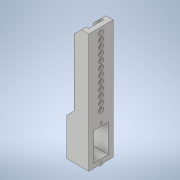
# Autodesk Inventor part: TopRearLeg4
Saved by Autodesk Inventor 2020 (Build 240168000, 168)
## iProperties
Created: 2019-03-31
Part Number: TopRearLeg4
Material: Generic
Document SubType Name: Modeling
Designer: cnam
Density: 1 g/cm^3
Appearance: Default
Author: cnam
Autodesk Inventor part; units mm, degrees
ref_plane "YZ Plane" through (0, 0, 0) normal (1, 0, 0) x (0, 1, 0)
ref_plane "XZ Plane" through (0, 0, 0) normal (0, 1, 0) x (-1, 0, 0)
ref_plane "XY Plane" through (0, 0, 0) normal (0, 0, 1) x (1, 0, 0)
sketch "Sketch1" plane through (0, 0, 0) normal (1, 0, 0) x (0, 1, 0)
  line L0 (47.75, -10) -> (-47.75, -10)
  line L1 (-47.75, -10) -> (-47.75, 10)
  line L2 (-47.75, 10) -> (47.75, 10)
  line L3 (47.75, 10) -> (47.75, -10)
  line L4 (47.75, -10) -> (-47.75, 10) construction
  line L5 (-47.75, -10) -> (47.75, 10) construction
  circle A0 centre (40.75, 0) radius 2
  circle A1 centre (-4.25, 0) radius 2
  line L6 (18.25, 25.1028) -> (18.25, -34.7635) construction
  line L7 (-1.75, 23.8417) -> (-1.75, -36.7999) construction
  circle A2 centre (20.75, 0) radius 2
  circle A3 centre (-24.25, 0) radius 2
  line L8 (-41.75, 23.8417) -> (-41.75, -30.9921) construction
  circle A4 centre (34.0833, 0) radius 2
  circle A5 centre (27.4167, 0) radius 2
  circle A6 centre (-10.9167, 0) radius 2
  circle A7 centre (-17.5833, 0) radius 2
  point P0 (0, 0)
  dimension "d1" = 20
  dimension "d4" = 4
  dimension "d5" = 7
  dimension "d6" = 45
  dimension "d7" = 22.5
  dimension "d8" = 20
  dimension "d9" = 22.5
  dimension "d10" = 22.5
  dimension "d11" = 60
  dimension "d18" = 6.6667
  dimension "d25" = 6.6667
  dimension "d30" = 6
  constraints: 18 end point, 8 centre point, 3 equal radius, 3 horizontal, 3 vertical, 2 midpoint, 2 parallel, 1 perpendicular, 8 other
  measures "d1" distance of L2.end L0.start
  measures "d4" diameter of A0
  measures "d5" distance from line of L3 A0.centre
  measures "d6" distance of A1.centre A0.centre
  measures "d7" distance from line of L6 A0.centre
  measures "d8" distance between parallel lines of L6 L7
  measures "d9" distance from line of L7 A2.centre
  measures "d10" distance from line of L7 A3.centre
  measures "d11" distance between parallel lines of L8 L6
  measures "d18" distance of A0.centre A4.centre
  measures "d25" distance of A1.centre A6.centre
  measures "d30" distance between parallel lines of L8 L1
extrude "Extrusion1" add sketch "Sketch1" along normal blind 4
sketch "Sketch2" plane through (0, 0, 0) normal (1, 0, 0) x (0, 1, 0)
  line L0 (-41.75, 22.3574) -> (-41.75, -36.9148) construction
  circle A0 centre (-17.5833, 0) radius 2 projected
  circle A1 centre (-10.9167, 0) radius 2 projected
  circle A2 centre (27.4167, 0) radius 2 projected
  circle A3 centre (34.0833, 0) radius 2 projected
  circle A4 centre (-24.25, 0) radius 2 projected
  circle A5 centre (20.75, 0) radius 2 projected
  circle A6 centre (-4.25, 0) radius 2 projected
  circle A7 centre (40.75, 0) radius 2 projected
  line L1 (-47.75, -10) -> (47.75, -10) projected
  line L2 (47.75, -10) -> (47.75, 10) projected
  line L3 (47.75, 10) -> (-47.75, 10) projected
  line L4 (-47.75, 10) -> (-47.75, -10) projected
  line L5 (47.75, 0) -> (-47.75, 0) construction
  line L6 (-47.75, -10) -> (-47.75, 10) projected
  line L7 (-59.75, -6.125) -> (-36.75, -6.125)
  line L8 (-36.75, -6.125) -> (-36.75, 6.125)
  line L9 (-36.75, 6.125) -> (-59.75, 6.125)
  line L10 (-59.75, 6.125) -> (-59.75, -6.125)
  line L11 (-59.75, -6.125) -> (-36.75, 6.125) construction
  line L12 (-36.75, -6.125) -> (-59.75, 6.125) construction
  line L13 (-47.75, -10) -> (-63.625, -10)
  line L14 (-63.625, -10) -> (-63.625, 10)
  line L15 (-63.625, 10) -> (-47.75, 10)
  line L16 (-47.75, 10) -> (-47.75, -10)
  line L17 (-32.875, -10) -> (-32.875, 10)
  point P0 (0, 0)
  point P1 (-48.25, 0)
  dimension "d33" = 6
  dimension "d34" = 12.25
  dimension "d35" = 23
  dimension "d36" = 5
  dimension "d37" = 3.875
  dimension "d38" = 3.875
  dimension "d39" = 3.875
  constraints: 26 end point, 4 midpoint, 4 parallel, 3 perpendicular, 3 point on line, 2 horizontal, 1 vertical
  measures "d33" distance between parallel lines of L4 L0
  measures "d34" distance of L7.end L8.end
  measures "d35" distance of L7.start L7.end
  measures "d36" distance between parallel lines of L0 L8
  measures "d37" distance between parallel lines of L15 L9
  measures "d38" distance between parallel lines of L14 L10
  measures "d39" distance between parallel lines of L8 L17
extrude "Extrusion2" cut sketch "Sketch2" along normal blind 20 contours L7 L10 L9 L4 | L4 L9 L8 L7
sketch "Sketch3" plane through (0, 0, 0) normal (-1, 0, 0) x (0, 0, 1)
  line L0 (-10, -47.75) -> (-6.125, -47.75) projected
  line L1 (-10, -47.75) -> (-6.125, -47.75)
  line L2 (6.125, -47.75) -> (10, -47.75) projected
  line L3 (10, -47.75) -> (6.125, -47.75)
  line L4 (6.125, -36.75) -> (6.125, -47.75) projected
  line L5 (6.125, -47.75) -> (10, -47.75) projected
  line L6 (10, -47.75) -> (10, 47.75) projected
  line L7 (10, 47.75) -> (-10, 47.75) projected
  line L8 (-10, 47.75) -> (-10, -47.75) projected
  line L9 (-10, -47.75) -> (-6.125, -47.75) projected
  line L10 (-6.125, -47.75) -> (-6.125, -36.75) projected
  line L11 (-6.125, -36.75) -> (6.125, -36.75) projected
  circle A0 centre (0, -17.5833) radius 2 projected
  circle A1 centre (0, -10.9167) radius 2 projected
  circle A2 centre (0, 27.4167) radius 2 projected
  circle A3 centre (0, 34.0833) radius 2 projected
  circle A4 centre (0, -24.25) radius 2 projected
  circle A5 centre (0, 20.75) radius 2 projected
  circle A6 centre (0, -4.25) radius 2 projected
  circle A7 centre (0, 40.75) radius 2 projected
  line L12 (-6.125, -36.75) -> (6.125, -36.75)
  line L13 (6.125, -36.75) -> (6.125, -59.75)
  line L14 (6.125, -59.75) -> (-6.125, -59.75)
  line L15 (-6.125, -59.75) -> (-6.125, -36.75)
  line L16 (-10, 47.75) -> (-10, -47.75) projected
  line L17 (-10, -32.875) -> (10, -32.875)
  line L18 (10, -32.875) -> (10, -63.625)
  line L19 (10, -63.625) -> (-10, -63.625)
  line L20 (-10, -63.625) -> (-10, -32.875)
  point P0 (0, 0)
  dimension "d44" = 23
  dimension "d45" = 3.875
  dimension "d46" = 3.875
  dimension "d47" = 3.875
  constraints: 20 end point, 5 equal length, 3 horizontal, 2 perpendicular, 1 point on line
  measures "d44" distance of L12.end L13.end
  measures "d45" distance between parallel lines of L12 L17
  measures "d46" distance between parallel lines of L19 L14
  measures "d47" distance between parallel lines of L18 L13
extrude "Extrusion4" add sketch "Sketch3" along normal blind 20 contours L8 L17 L6 L2 L4 L11 L10 L0 | L0 L15 L14 L13 L2 L18 L19 L20
sketch "Sketch5" plane through (0, 0, 0) normal (1, 0, 0) x (0, 0, -1)
  line L0 (-6.125, -47.75) -> (-10, -47.75) projected
  line L1 (-10, -63.625) -> (-10, -47.75) projected
  line L2 (10, -63.625) -> (-10, -63.625) projected
  line L3 (10, -47.75) -> (10, -63.625) projected
  line L4 (10, -47.75) -> (6.125, -47.75) projected
  line L5 (6.125, -47.75) -> (6.125, -59.75) projected
  line L6 (6.125, -59.75) -> (-6.125, -59.75) projected
  line L7 (-6.125, -59.75) -> (-6.125, -47.75) projected
  point P0 (0, 0)
extrude "Extrusion5" add sketch "Sketch5" along normal blind 4
sketch "Sketch6" plane through (0, 0, 0) normal (-1, 0, 0) x (0, 0, 1)
  line L0 (-10, -32.875) -> (10, -32.875) projected
  line L1 (10, -32.875) -> (10, 47.75) projected
  line L2 (10, 47.75) -> (-10, 47.75) projected
  line L3 (-10, 47.75) -> (-10, -32.875) projected
  circle A0 centre (0, -17.5833) radius 2 projected
  circle A1 centre (0, -10.9167) radius 2 projected
  circle A2 centre (0, 27.4167) radius 2 projected
  circle A3 centre (0, 34.0833) radius 2 projected
  circle A4 centre (0, -24.25) radius 2 projected
  circle A5 centre (0, 20.75) radius 2 projected
  circle A6 centre (0, -4.25) radius 2 projected
  circle A7 centre (0, 40.75) radius 2 projected
  circle A8 centre (0, -30.375) radius 0.875
  point P0 (0, 0)
  dimension "d52" = 2.5
  dimension "d53" = 1.75
  constraints: 1 centre point
  measures "d52" distance from line of L0 A8.centre
  measures "d53" diameter of A8
extrude "Extrusion6" cut sketch "Sketch6" against normal blind 4 contours A8
sketch "Sketch8" plane through (4, 47.75, -10) normal (0, 0, -1) x (-1, 0, 0)
  line L0 (24, -84.5) -> (0, -84.5) projected
  line L1 (4, 0) -> (4, -80.625) projected
  line L2 (4, 0) -> (0, 0) projected
  line L3 (0, -111.375) -> (0, 0) projected
  line L4 (0, -111.375) -> (24, -111.375) projected
  line L5 (24, -80.625) -> (24, -111.375) projected
  line L6 (4, -80.625) -> (24, -80.625) projected
  line L7 (4, -80.625) -> (4, 0) projected
  line L8 (4, 0) -> (4, -80.625) projected
  line L9 (24, -80.625) -> (4, 0)
  point P0 (4, -47.75)
  constraints: 2 end point
extrude "Extrusion8" add sketch "Sketch8" against normal blind 3 contours L6 L1 L9
mirror "Mirror2" about plane through (0, 0, 0) normal (0, 0, 1) of "Extrusion8"
sketch "Sketch9" plane through (4, 0, 0) normal (1, 0, 0) x (0, 0, -1)
  circle A0 centre (0, -30.375) radius 0.875 projected
  line L0 (10, -63.625) -> (10, 47.75) projected
  line L1 (10, 47.75) -> (-10, 47.75) projected
  line L2 (-10, 47.75) -> (-10, -63.625) projected
  line L3 (-10, -63.625) -> (10, -63.625) projected
  line L4 (6.125, -36.75) -> (6.125, -59.75) projected
  line L5 (6.125, -59.75) -> (-6.125, -59.75) projected
  line L6 (-6.125, -59.75) -> (-6.125, -36.75) projected
  line L7 (-6.125, -36.75) -> (6.125, -36.75) projected
  circle A1 centre (0, 40.75) radius 2 projected
  circle A2 centre (0, -4.25) radius 2 projected
  circle A3 centre (0, 20.75) radius 2 projected
  circle A4 centre (0, -24.25) radius 2 projected
  circle A5 centre (0, 34.0833) radius 2 projected
  circle A6 centre (0, 27.4167) radius 2 projected
  circle A7 centre (0, -10.9167) radius 2 projected
  circle A8 centre (0, -17.5833) radius 2 projected
  point P0 (0, 0)
sketch "Sketch10" plane through (0, 0, 0) normal (-1, 0, 0) x (0, 0, 1)
  line L0 (-3.7215, 44.8818) -> (4.317, 44.8818)
  line L1 (4.317, 44.8818) -> (4.317, -27.7627)
  line L2 (4.317, -27.7627) -> (-3.7215, -27.7627)
  line L3 (-3.7215, -27.7627) -> (-3.7215, 44.8818)
  point P0 (0, 0)
  constraints: 8 end point, 2 parallel, 1 horizontal, 1 perpendicular
extrude "Extrusion9" add sketch "Sketch10" against normal blind 4
sketch "Sketch11" plane through (0, 0, 0) normal (-1, 0, 0) x (0, 0, 1)
  circle A0 centre (0, -30.375) radius 0.875 projected
  line L0 (7, -32.875) -> (7, 47.75) projected
  line L1 (7, 47.75) -> (-7, 47.75) projected
  line L2 (-7, 47.75) -> (-7, -32.875) projected
  line L3 (-7, -32.875) -> (7, -32.875) projected
  arc A1 (2, -30.375) -> (-2, -30.375) centre (0, -30.375) ccw
  line L4 (-7, -32.875) -> (7, -32.875) projected
  line L5 (-0.875, -30.375) -> (0.875, -30.375)
  line L6 (2, -30.375) -> (2, -32.875)
  line L7 (2, -32.875) -> (-2, -32.875)
  line L8 (-2, -32.875) -> (-2, -30.375)
  point P0 (0, 0)
  point P1 (-2, -32.875)
  dimension "d68" = 4
  constraints: 8 end point, 4 point on circle, 2 parallel, 1 centre point, 1 coincident, 1 horizontal, 1 perpendicular, 1 point on line
  measures "d68" diameter of A1
extrude "Extrusion10" add sketch "Sketch11" along normal blind 20 contours L3 L8 A1 L6
sketch "Sketch12" plane through (0, 0, 0) normal (-1, 0, 0) x (0, 0, 1)
  line L0 (2, -30.375) -> (2, -32.875) projected
  line L1 (2, -32.875) -> (7, -32.875) projected
  line L2 (7, -32.875) -> (7, 47.75) projected
  line L3 (7, 47.75) -> (-7, 47.75) projected
  line L4 (-7, 47.75) -> (-7, -32.875) projected
  line L5 (-7, -32.875) -> (-2, -32.875) projected
  line L6 (-2, -32.875) -> (-2, -30.375) projected
  arc A0 (2, -30.375) -> (-2, -30.375) centre (0, -30.375) ccw projected
  point P0 (0, 0)
  point P1 (0, 44.75)
  point P2 (0, 39.75)
  point P3 (0, 34.75)
  point P4 (0, 29.75)
  point P5 (0, 24.75)
  point P6 (0, 19.75)
  point P7 (0, 14.75)
  point P8 (0, 9.75)
  point P9 (0, 4.75)
  point P10 (0, -0.25)
  point P11 (0, -5.25)
  point P12 (0, -10.25)
  point P13 (0, -15.25)
  point P14 (0, -20.25)
  point P15 (0, -25.25)
  dimension "d74" = 5
  constraints: 1 vertical, 14 other
  measures "d74" distance of point (0, 44.75) point (0, 39.75)
hole "Hole1" at (0, 44.75, 0) at (0, 39.75, 0) at (0, 34.75, 0) at (0, 29.75, 0) at (0, 24.75, 0) at (0, 19.75, 0) at (0, 14.75, 0) at (0, 9.75, 0) at (0, 4.75, 0) at (0, -0.25, 0) at (0, -5.25, 0) at (0, -10.25, 0) at (0, -15.25, 0) at (0, -20.25, 0) at (0, -25.25, 0) direction (1, 0, 0) diameter 4 end through all
sketch "Sketch13" plane through (-20, 0, 0) normal (-1, 0, 0) x (0, 0, 1)
  line L0 (-19.5017, -86.8207) -> (19.9399, -86.8207)
  line L1 (19.9399, -86.8207) -> (19.9399, 61.3045)
  line L2 (19.9399, 61.3045) -> (-19.5017, 61.3045)
  line L3 (-19.5017, 61.3045) -> (-19.5017, -86.8207)
  point P0 (0, 0)
  constraints: 8 end point, 2 parallel, 1 horizontal, 1 perpendicular
extrude "Extrusion11" cut sketch "Sketch13" against normal blind 6
sketch "Sketch14" plane through (-14, 0, 0) normal (-1, 0, 0) x (0, 0, 1)
  line L0 (6.125, -59.75) -> (6.125, -36.75) projected
  line L1 (6.125, -59.75) -> (6.125, -36.75) projected
  line L2 (6.125, -48.25) -> (-6.125, -48.25)
  line L3 (-6.125, -36.75) -> (-6.125, -59.75) projected
  point P0 (0, 0)
  constraints: 2 end point, 2 midpoint
surface extrude "ExtrusionSrf1" sketch "Sketch14" against normal mid plane 50 shown no curves L2
mirror "Mirror3" about plane through (-14, -48.25, 6.125) normal (0, -1, 0) of "Extrusion10"
sketch "Sketch15" plane through (-20, -66.125, -2) normal (-1, 0, 0) x (0, 0, 1)
  circle A0 centre (2, 0) radius 0.875 projected
  line L0 (0, 0) -> (0, 2.5) projected
  arc A1 (0, 0) -> (4, 0) centre (2, 0) ccw projected
  line L1 (4, 2.5) -> (4, 0) projected
  line L2 (0, 2.5) -> (4, 2.5) projected
  circle A2 centre (2, 0) radius 0.875 projected
  point P0 (2, 66.125)
extrude "Extrusion12" cut sketch "Sketch15" against normal up to surface (6 mm away) contours A0 | L0 L2 L1 A1
sketch "Sketch16" plane through (0, -66.125, -2) normal (1, 0, 0) x (0, 0, -1)
  line L0 (0, 0) -> (0, 2.5) projected
  line L1 (-4, 2.5) -> (0, 2.5) projected
  line L2 (-4, 2.5) -> (-4, 0) projected
  arc A0 (-4, 0) -> (0, 0) centre (-2, 0) ccw projected
  circle A1 centre (-2, 0) radius 0.875 projected
  point P0 (-2, 66.125)
extrude "Extrusion13" add sketch "Sketch16" along normal up to surface (4 mm away)
chamfer "Chamfer1" distance 16 angle 45 2 edges at (-14, -8.6875, -8.5) (-14, -8.6875, 8.5)
sketch "Sketch17" plane through (-14, 0, 0) normal (-1, 0, 0) x (0, 0, 1)
  circle A0 centre (0, -66.125) radius 0.875 projected
  circle A1 centre (0, -30.375) radius 0.875 projected
  line L0 (7, -24.6875) -> (10, -24.6875) projected
  line L1 (7, -32.875) -> (7, -24.6875) projected
  line L2 (2, -32.875) -> (7, -32.875) projected
  line L3 (2, -30.375) -> (2, -32.875) projected
  arc A2 (2, -30.375) -> (-2, -30.375) centre (0, -30.375) ccw projected
  line L4 (-2, -32.875) -> (-2, -30.375) projected
  line L5 (-7, -32.875) -> (-2, -32.875) projected
  line L6 (-7, -24.6875) -> (-7, -32.875) projected
  line L7 (-10, -24.6875) -> (-7, -24.6875) projected
  line L8 (-10, -63.625) -> (-10, -24.6875) projected
  line L9 (-2, -63.625) -> (-10, -63.625) projected
  line L10 (-2, -66.125) -> (-2, -63.625) projected
  arc A3 (-2, -66.125) -> (2, -66.125) centre (0, -66.125) ccw projected
  line L11 (2, -63.625) -> (2, -66.125) projected
  line L12 (10, -63.625) -> (2, -63.625) projected
  line L13 (10, -24.6875) -> (10, -63.625) projected
  line L14 (6.125, -36.75) -> (-6.125, -36.75) projected
  line L15 (6.125, -59.75) -> (6.125, -36.75) projected
  line L16 (-6.125, -59.75) -> (6.125, -59.75) projected
  line L17 (-6.125, -36.75) -> (-6.125, -59.75) projected
  line L18 (-7, -24.6875) -> (-7, -32.875) projected
  line L19 (-7, -32.875) -> (-26.1953, -32.875)
  line L20 (-26.1953, -32.875) -> (-26.1953, 59.8507)
  line L21 (-26.1953, 59.8507) -> (-7, 59.8507)
  line L22 (-7, 59.8507) -> (-7, -32.875)
  line L23 (2, -32.875) -> (7, -32.875) projected
  line L24 (7, -32.875) -> (27.7212, -32.875)
  line L25 (27.7212, -32.875) -> (27.7212, 59.8507)
  line L26 (27.7212, 59.8507) -> (7, 59.8507)
  line L27 (7, 59.8507) -> (7, -32.875)
  point P0 (0, 0)
  constraints: 16 end point, 4 parallel, 2 horizontal, 2 perpendicular, 1 point on line
extrude "Extrusion14" cut sketch "Sketch17" against normal up to surface (14 mm away) contours L27 L26 L25 L24 L13 L0 | L0 L13 L24 L1 | L19 L8 L7 L6 | L7 L8 L19 L20 L21 L22
sketch "Sketch18" plane through (0, 47.75, 10) normal (0, 0, 1) x (1, 0, 0)
  line L0 (0, 0) -> (0, -80.625) projected
  line L1 (0, -80.625) -> (-14, -80.625) projected
  line L2 (-14, -80.625) -> (-14, -111.375) projected
  line L3 (4, -111.375) -> (-14, -111.375) projected
  line L4 (4, 0) -> (4, -111.375) projected
  line L5 (0, 0) -> (4, 0) projected
  line L6 (-14, -80.625) -> (0, -80.625) projected
  line L7 (-14, -80.625) -> (0, -66.625)
  point P0 (0, -47.75)
  dimension "d101" = 45
  constraints: 2 end point, 1 point on line
  measures "d101" angle of L1 L7
extrude "Extrusion15" add sketch "Sketch18" against normal blind 4 contours L0 L1 L7
sketch "Sketch19" plane through (0, 0, 0) normal (-1, 0, 0) x (0, 0, 1)
  line L0 (10, 47.75) -> (10, -63.625) projected
  line L1 (6, -32.875) -> (2, -32.875) projected
  line L2 (10, 47.75) -> (6, 47.75)
  line L3 (6, 47.75) -> (6, -32.875)
  line L4 (6, -32.875) -> (10, -32.875)
  line L5 (10, -32.875) -> (10, 47.75)
  point P0 (0, 0)
  constraints: 8 end point, 2 parallel, 1 horizontal, 1 perpendicular
extrude "Extrusion16" add sketch "Sketch19" along normal blind 8
chamfer "Chamfer2" distance 8 angle 45 1 edges at (-8, 47.75, 8)
mirror "Mirror4" about plane through (0, 0, 0) normal (0, 0, 1) of "Extrusion15", "Extrusion16", "Chamfer2"
fillet "Fillet4" radius 4 2 edges at (2, 47.75, 10) (2, 47.75, -10)
fillet "Fillet5" radius 4 2 edges at (-8, 39.75, -8) (-8, 39.75, 8)
sketch "Sketch20" plane through (-14, 0, 0) normal (-1, 0, 0) x (0, 0, 1)
  line L0 (6.125, -36.75) -> (-6.125, -36.75) projected
  line L1 (-6.125, -59.75) -> (6.125, -59.75) projected
  point P0 (0, 0)
  point P1 (0, -34.25)
  point P2 (0, -62.25)
  dimension "d111" = 2.5
  dimension "d112" = 2.5
  measures "d111" distance from line of L0 point (0, -34.25)
  measures "d112" distance from line of point (0, -62.25) L1
hole "Hole2" at (-14, -34.25, 0) at (-14, -62.25, 0) direction (1, 0, 0) diameter 1.75 end through all
sketch "Sketch21" plane through (-14, 0, 0) normal (-1, 0, 0) x (0, 0, 1)
  circle A0 centre (0, -34.25) radius 0.875 projected
  circle A1 centre (0, -62.25) radius 0.875 projected
  line L0 (10, -32.875) -> (6, -32.875) projected
  line L1 (6, -32.875) -> (2, -32.875) projected
  line L2 (2, -30.375) -> (2, -32.875) projected
  arc A2 (2, -30.375) -> (-2, -30.375) centre (0, -30.375) ccw projected
  line L3 (-2, -32.875) -> (-2, -30.375) projected
  line L4 (-2, -32.875) -> (-6, -32.875) projected
  line L5 (-6, -32.875) -> (-10, -32.875) projected
  line L6 (-10, -63.625) -> (-10, -32.875) projected
  line L7 (-2, -63.625) -> (-10, -63.625) projected
  line L8 (-2, -66.125) -> (-2, -63.625) projected
  arc A3 (-2, -66.125) -> (2, -66.125) centre (0, -66.125) ccw projected
  line L9 (2, -63.625) -> (2, -66.125) projected
  line L10 (10, -63.625) -> (2, -63.625) projected
  line L11 (10, -32.875) -> (10, -63.625) projected
  line L12 (6.125, -36.75) -> (-6.125, -36.75) projected
  line L13 (6.125, -59.75) -> (6.125, -36.75) projected
  line L14 (-6.125, -59.75) -> (6.125, -59.75) projected
  line L15 (-6.125, -36.75) -> (-6.125, -59.75) projected
  circle A4 centre (0, -30.375) radius 0.875 projected
  circle A5 centre (0, -66.125) radius 0.875 projected
  line L16 (-2, -63.625) -> (2, -63.625)
  line L17 (6, -32.875) -> (2, -32.875) projected
  line L18 (2, -32.875) -> (-2, -32.875)
  point P0 (0, 0)
  constraints: 4 end point, 1 collinear, 1 horizontal
extrude "Extrusion17" cut sketch "Sketch21" against normal up to surface (14 mm away) contours L18 L3 A2 L2 | L9 A3 L8 L16
sketch "Sketch22" plane through (0, -66.125, -2) normal (-1, 0, 0) x (0, 0, 1)
  circle A0 centre (2, 0) radius 0.875 projected
  line L0 (4, 2.5) -> (0, 2.5) projected
  line L1 (0, 0) -> (0, 2.5) projected
  arc A1 (0, 0) -> (4, 0) centre (2, 0) ccw projected
  line L2 (4, 2.5) -> (4, 0) projected
  point P0 (2, 66.125)
extrude "Extrusion18" cut sketch "Sketch22" against normal blind 10 contours A0 | L2 A1 L1 L0
sketch "Sketch23" plane through (0, 0, 0) normal (-1, 0, 0) x (0, 0, 1)
  circle A0 centre (0, -30.375) radius 0.875 projected
  point P0 (0, 0)
extrude "Extrusion19" add sketch "Sketch23" against normal blind 4
sketch "Sketch24" plane through (-14, 0, 0) normal (-1, 0, 0) x (0, 0, 1)
  line L0 (10, -63.625) -> (-10, -63.625) projected
  line L1 (10, -32.875) -> (10, -63.625) projected
  line L2 (10, -32.875) -> (6, -32.875) projected
  line L3 (6, -32.875) -> (-6, -32.875) projected
  line L4 (-6, -32.875) -> (-10, -32.875) projected
  line L5 (-10, -63.625) -> (-10, -32.875) projected
  circle A0 centre (0, -34.25) radius 0.875 projected
  circle A1 centre (0, -62.25) radius 0.875 projected
  line L6 (6.125, -36.75) -> (-6.125, -36.75) projected
  line L7 (6.125, -59.75) -> (6.125, -36.75) projected
  line L8 (-6.125, -59.75) -> (6.125, -59.75) projected
  line L9 (-6.125, -36.75) -> (-6.125, -59.75) projected
  circle A2 centre (0, -34.25) radius 0.875 projected
  circle A3 centre (0, -34.25) radius 2.5
  circle A4 centre (0, -62.25) radius 2.5
  point P0 (0, 0)
  point P1 (-2.0879, -32.875)
  point P2 (2.0879, -32.875)
  point P3 (-2.0879, -63.625)
  point P4 (2.0879, -63.625)
  constraints: 2 centre point, 2 coincident
extrude "Extrusion20" add sketch "Sketch24" against normal up to surface (18 mm away) contours A4 L0 | L3 A3 picked at (-0.2038, -63.9747) picked at (-0.2038, -32.2127)
sketch "Sketch25" plane through (0, 0, 0) normal (-1, 0, 0) x (0, 0, 1)
  circle A0 centre (0, 34.75) radius 2 projected
  circle A1 centre (0, 39.75) radius 2 projected
  circle A2 centre (0, 44.75) radius 2 projected
  point P0 (0, 0)
extrude "Extrusion21" add sketch "Sketch25" against normal up to surface (4 mm away)
sketch "Sketch26" plane through (0, 0, 0) normal (-1, 0, 0) x (0, 0, 1)
  line L0 (-17.4187, 33.75) -> (21.8321, 33.75)
  line L1 (21.8321, 33.75) -> (21.8321, 58.5819)
  line L2 (21.8321, 58.5819) -> (-17.4187, 58.5819)
  line L3 (-17.4187, 58.5819) -> (-17.4187, 33.75)
  circle A0 centre (0, 29.75) radius 2 projected
  point P0 (0, 0)
  dimension "d130" = 4
  constraints: 8 end point, 2 parallel, 1 horizontal, 1 perpendicular
  measures "d130" distance from line of L0 A0.centre
extrude "Extrusion22" cut sketch "Sketch26" along normal blind 10 and the other way blind 5 contours L3 L2 L1 L0
chamfer "Chamfer3" distance 6 angle 45 2 edges at (-8, 33.75, -8) (-8, 33.75, 8)
body "Solid1"
body "Srf1"
